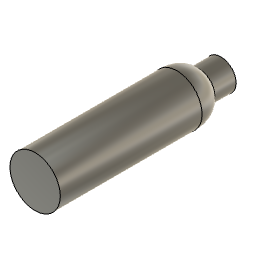
bottle (Autodesk Fusion 360 design; units mm, degrees)
Autodesk Fusion 360 part; units mm, degrees
sketch "Sketch1" plane through (0, 0, 0) normal (0, 0, 1) x (1, 0, 0)
  line L0 (0, 0) -> (0, 262)
  line L1 (0, 262) -> (-21.525, 262)
  line L2 (-21.525, 262) -> (-21.525, 231.82)
  line L3 (-21.525, 231.82) -> (0, 231.82)
  line L4 (0, 0) -> (-35.485, 0)
  line L5 (-35.485, 0) -> (-35.485, 200)
  spline S0 degree 5 poles (-35.485, 200) (-35.4774, 200.8274) (-35.439, 202.4658) (-35.3116, 204.8744) (-34.9997, 207.9859) (-34.3566, 211.6973) (-33.4363, 215.2138) (-32.2139, 218.5178) (-30.6718, 221.5971) (-28.8168, 224.4564) (-26.6703, 227.1107) (-24.7378, 229.0827) (-23.1749, 230.4819) (-22.0832, 231.3798) (-21.525, 231.82) knots 0 0 0 0 0 0 0.1 0.2 0.3 0.4 0.5 0.6 0.7 0.8 0.9 1 1 1 1 1 1
  point P0 (-31.849, 219.1008)
  dimension "d2" = 262
  dimension "d6" = 21.525
  dimension "d7" = 30.18
  dimension "d8" = 35.485
  constraint coincident L0.start L4.start
  constraint vertical L0
  constraint perpendicular L0 L1
  constraint perpendicular L1 L2
  constraint coincident L0 L3.end
  constraint perpendicular L0 L3
  constraint perpendicular L0 L4
  constraint perpendicular L4 L5
  measures "d2" distance of L0.start L0.end
  measures "d6" distance of L0.end L1.end
  measures "d7" distance of L1.end L2.end
  measures "d8" distance of L0.start L4.end
revolve "Revolve1" add sketch "Sketch1" angle 360 about axis through (0, 0, 0) along (0, 1, 0)
equation "diameter = 70.97 mm"
equation "d2 = bottle_length"
equation "bottle_length = 262 mm"
equation "cap_diameter = 43.05 mm"
equation "cap_length = 30.18 mm"
equation "d6 = cap_diameter / 2"
equation "d7 = cap_length"
equation "d8 = bottle_diameter / 2"
equation "bottle_diameter = 70.97 mm"
